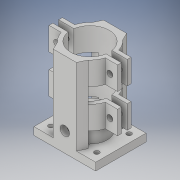
# Autodesk Inventor part: Mount
Saved by Autodesk Inventor 2018 (Build 220112000, 112)
## iProperties
Created: 2018-03-27
Part Number: Mount
Material: Generic
Document SubType Name: Modeling
Designer: prakh
Density: 1 g/cm^3
Appearance: Default
Author: prakh
Autodesk Inventor part; units mm, degrees
ref_plane "YZ Plane" through (0, 0, 0) normal (1, 0, 0) x (0, 1, 0)
ref_plane "XZ Plane" through (0, 0, 0) normal (0, 1, 0) x (-1, 0, 0)
ref_plane "XY Plane" through (0, 0, 0) normal (0, 0, 1) x (1, 0, 0)
sketch "Sketch1" plane through (0, 0, 0) normal (0, 1, 0) x (-1, 0, 0)
  line L0 (25.527, 20.828) -> (-25.527, 20.828)
  line L1 (-25.527, 20.828) -> (-25.527, -20.828)
  line L2 (-25.527, -20.828) -> (25.527, -20.828)
  line L3 (25.527, -20.828) -> (25.527, 20.828)
  circle A0 centre (18.9992, 13.3858) radius 1.9837
  circle A1 centre (18.9992, -13.3858) radius 1.9837
  circle A2 centre (-18.9992, -13.3858) radius 1.9837
  circle A3 centre (-18.9992, 13.3858) radius 1.9837
  circle A4 centre (18.9992, 13.3858) radius 3.048 construction
  point P0 (0, 0)
  point P1 (25.527, 0)
  point P2 (0, -20.828)
  dimension "d0" = 3.9675
  dimension "d1" = 41.656
  dimension "d2" = 51.054
  dimension "d3" = 6.096
  dimension "d4" = 7.4422
  dimension "d5" = 6.5278
  dimension "d6" = 7.4422
  dimension "d7" = 6.5278
  constraints: 8 end point, 5 centre point, 3 equal radius, 3 horizontal alignment, 3 vertical alignment, 2 midpoint, 2 parallel, 1 coincident, 1 horizontal, 1 perpendicular
  measures "d0" diameter of A1
  measures "d1" distance of L2.end L0.start
  measures "d2" distance of L0.start L0.end
  measures "d3" diameter of A4
  measures "d4" distance from line of L0 A4.centre
  measures "d5" distance from line of A4.centre L3
  measures "d6" distance from line of L2 A2.centre
  measures "d7" distance from line of A2.centre L1
extrude "Extrusion1" add sketch "Sketch1" along normal blind 6.35
ref_plane "Work Plane1" through (0, 69.85, 0) normal (0, 1, 0) x (1, 0, 0)
sketch "Sketch3" plane through (0, 6.35, 0) normal (0, 1, 0) x (1, 0, 0)
  line L0 (-28.3954, -5.5563) -> (-28.3954, -2.3813)
  line L1 (28.3954, -2.3812) -> (28.3954, -5.5563)
  line L2 (28.3954, -5.5563) -> (18.2217, -5.5563)
  line L3 (-18.2217, -5.5563) -> (-28.3954, -5.5563)
  line L4 (-28.3954, -2.3813) -> (-15.6954, -2.3813)
  line L5 (15.6954, -2.3812) -> (28.3954, -2.3812)
  arc A0 (-18.2217, -5.5563) -> (18.2217, -5.5563) centre (0, 0) ccw
  arc A1 (-15.6954, -2.3813) -> (15.6954, -2.3812) centre (0, 0) ccw
  line L6 (-25.527, -20.828) -> (25.527, -20.828) projected
  line L7 (9.525, -20.828) -> (-9.525, -20.828)
  line L8 (-25.527, -20.828) -> (25.527, -20.828) projected
  line L9 (-9.525, -20.828) -> (-12.7, -14.199)
  line L10 (9.525, -20.828) -> (12.7, -14.199)
  dimension "d26" = 15.875
  dimension "d27" = 3.175
  dimension "d28" = 3.175
  dimension "d29" = 3.175
  dimension "d30" = 2.3813
  dimension "d31" = 2.3813
  dimension "d32" = 19.05
  dimension "d33" = 9.525
  dimension "d34" = 25.4
  dimension "d43" = 12.7
  dimension "d44" = 12.7
  constraints: 18 end point, 6 point on circle, 5 parallel, 2 centre point, 2 coincident, 2 horizontal, 2 perpendicular, 2 point on line, 1 equal length
  measures "d26" radius of A1
  measures "d27" radial gap between concentric circles of A1 A0
  measures "d28" distance between parallel lines of L5 L2
  measures "d29" distance between parallel lines of L3 L4
  measures "d30" distance from line of point (0, 0) L4
  measures "d31" distance from line of point (0, 0) L5
  measures "d32" distance of L7.end L7.start
  measures "d33" horizontal distance of point (0, 0) L7.end
  measures "d34" distance of L9.end L10.end
  measures "d43" distance of L0.end L4.end
  measures "d44" distance of L5.start L1.start
extrude "Extrusion3" add sketch "Sketch3" along normal blind 63.5
sketch "Sketch6" plane through (25.527, 6.35, 2.3812) normal (0, 0, -1) x (-1, 0, 0)
  line L0 (0, 0) -> (7.3053, 0) projected
  line L1 (53.9224, 0) -> (53.9224, 63.5) projected
  line L2 (0, 0) -> (53.9224, 0)
  line L3 (53.9224, 0) -> (53.9224, 12.7)
  line L4 (53.9224, 12.7) -> (0, 12.7)
  line L5 (0, 12.7) -> (0, 0)
  line L6 (53.9224, 31.75) -> (0, 31.75)
  line L7 (0, 31.75) -> (0, 44.45)
  line L8 (0, 44.45) -> (53.9224, 44.45)
  line L9 (53.9224, 44.45) -> (53.9224, 31.75)
  line L10 (0, 44.45) -> (-2.8684, 44.45)
  line L11 (-2.8684, 44.45) -> (-2.8684, 31.75)
  line L12 (-2.8684, 31.75) -> (0, 31.75)
  line L13 (0, 31.75) -> (0, 44.45)
  line L14 (-2.8684, 0) -> (-2.8684, 63.5) projected
  line L15 (0, 12.7) -> (-2.8684, 12.7)
  line L16 (-2.8684, 12.7) -> (-2.8684, 0)
  line L17 (-2.8684, 0) -> (0, 0)
  line L18 (0, 0) -> (0, 12.7)
  line L19 (-2.8684, 0) -> (-2.8684, 63.5) projected
  line L20 (0, 0) -> (51.054, 0) projected
  point P0 (25.527, -6.35)
  point P1 (53.9224, 63.5)
  dimension "d37" = 12.7
  dimension "d38" = 12.7
  dimension "d39" = 19.05
  constraints: 32 end point, 8 parallel, 4 horizontal, 4 perpendicular, 3 collinear, 2 point on line, 3 other
  measures "d37" distance of L4.end L0.start
  measures "d38" distance of L6.end L7.end
  measures "d39" distance between parallel lines of L6 L4
extrude "Extrusion4" cut sketch "Sketch6" against normal up to surface (11.8178 mm away) contours L5 L4 L1 L2 L0 | L17 L14 L15 L5 | L6 L7 L8 L1 | L11 L10 L7 L12
sketch "Sketch7" plane through (28.3954, 69.85, 2.3812) normal (0, 0, -1) x (-1, 0, 0)
  circle A0 centre (50.4408, -9.525) radius 2.4575
  circle A1 centre (50.4408, -41.275) radius 2.4575
  circle A2 centre (6.35, -41.275) radius 2.4575
  circle A3 centre (6.35, -9.525) radius 2.4575
  line L0 (56.7908, -50.8) -> (56.7908, -31.75) projected
  line L1 (56.7908, -19.05) -> (56.7908, 0) projected
  line L2 (0, -19.05) -> (0, 0) projected
  line L3 (0, -50.8) -> (0, -31.75) projected
  point P0 (28.3954, -69.85)
  point P1 (56.7908, -41.275)
  point P2 (56.7908, -9.525)
  point P3 (0, -9.525)
  point P4 (0, -41.275)
  point P5 (56.7908, -9.525)
  dimension "d45" = 6.35
  dimension "d46" = 6.35
  dimension "d47" = 6.35
  dimension "d48" = 6.35
  dimension "d51" = 4.9149
  constraints: 5 midpoint, 4 centre point, 4 horizontal alignment, 3 equal radius
  measures "d45" distance from line of L2 A3.centre
  measures "d46" distance from line of A2.centre L3
  measures "d47" distance from line of A1.centre L0
  measures "d48" distance from line of A0.centre L1
  measures "d51" diameter of A0
extrude "Extrusion5" cut sketch "Sketch7" against normal blind 63.5
mirror "Mirror1" about plane through (0, 0, 0) normal (0, 0, 1) of "Extrusion3", "Extrusion5", "Extrusion4"
sketch "Sketch8" plane through (0, 6.35, 0) normal (0, 1, 0) x (1, 0, 0)
  circle A0 centre (0, 0) radius 14.351
  dimension "d52" = 28.702
  constraints: 1 centre point, 1 coincident
  measures "d52" diameter of A0
extrude "Extrusion6" add sketch "Sketch8" along normal blind 12.7
sketch "Sketch9" plane through (-25.527, 0, 20.828) normal (0, 0, 1) x (1, 0, 0)
  circle A0 centre (25.527, 16.0274) radius 3.937
  line L0 (0, 0) -> (51.054, 0) projected
  line L1 (35.052, 6.35) -> (51.054, 6.35) projected
  point P0 (25.527, 0)
  dimension "d55" = 7.874
  dimension "d57" = 9.6774
  constraints: 1 centre point
  measures "d55" diameter of A0
  measures "d57" distance from line of A0.centre L1
extrude "Extrusion7" cut sketch "Sketch9" against normal blind 61.9125
equation "\"d6\" = d4"
equation "\"d7\" = d5"
equation "\"d33\" = 0.5 * d32"
equation "\"d46\" = d45"
equation "\"d47\" = d45"
equation "\"d48\" = d45"
equation "\"d23\" = d22"
equation "\"d25\" = 0.5 * d24"
equation "\"d22\" = 3.175"
equation "\"d24\" = 4.7625"
body "Solid1"
